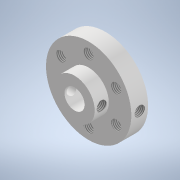
# Autodesk Inventor part: hub polulu
Saved by Autodesk Inventor 2020.3 (Build 243373000, 373)
## iProperties
Created: 2021-01-22
Part Number: hub polulu
Material: Generic
Document SubType Name: Modeling
Designer: Yu Jinyu
Density: 1 g/cm^3
Appearance: Default
Author: Yu Jinyu
Autodesk Inventor part; units mm, degrees
ref_plane "XZ Plane" through (0, 0, 0) normal (0, 1, 0) x (-1, 0, 0)
ref_plane "XY Plane" through (0, 0, 0) normal (0, 0, 1) x (1, 0, 0)
sketch "Sketch1" plane through (0, 0, 0) normal (0, 0, 1) x (1, 0, 0)
  circle A0 centre (0, 0) radius 12.7
  dimension "d0" = 25.4
  constraints: 1 centre point, 1 coincident
  measures "d0" diameter of A0
extrude "Extrusion1" add sketch "Sketch1" along normal blind 5
sketch "Sketch2" plane through (0, 0, 5) normal (0, 0, 1) x (1, 0, 0)
  circle A0 centre (0, 0) radius 6
  circle A1 centre (0, 0) radius 3
  dimension "d3" = 12
  dimension "d4" = 6
  constraints: 2 centre point, 2 coincident
  measures "d3" diameter of A0
  measures "d4" diameter of A1
extrude "Extrusion2" add sketch "Sketch2" along normal blind 4.2
sketch "Sketch3" plane through (0, 0, 5) normal (0, 0, 1) x (1, 0, 0)
  circle A0 centre (0, 0) radius 6 projected
  circle A1 centre (0, 0) radius 6
  circle A2 centre (0, 0) radius 9.5
  circle A3 centre (0, 9.5) radius 1.5
  circle A4 centre (0, 0) radius 3
  dimension "d7" = 19
  dimension "d8" = 3
  constraints: 3 centre point, 3 coincident, 1 vertical alignment, 2 other
  measures "d8" diameter of A3
extrude "Extrusion3" cut sketch "Sketch3" against normal blind 5 contours A3 A2 | A2 A3 | A4 picked at (0, 8.9912) picked at (0.0421, 9.9894)
pattern_circular "Circular Pattern1" count 6 over 360 about axis through (0, 0, 0) along (0, 0, 1) of "Extrusion1", "Extrusion3"
sketch "Sketch4" plane through (0, 0, 5) normal (0, 0, 1) x (1, 0, 0)
  circle A0 centre (0, 0) radius 9.5
  circle A1 centre (0, 9.5) radius 1.5
  dimension "d14" = 19
  dimension "d15" = 3
  constraints: 1 centre point, 1 coincident, 1 vertical alignment, 2 other
  measures "d15" diameter of A1
extrude "Extrusion4" cut sketch "Sketch4" against normal blind 10 contours A1 A0 | A0 A1 picked at (0, 8.9912) picked at (0.0421, 9.9894)
ref_plane "Work Plane1" through (12.7, 0, 0) normal (1, 0, 0) x (0, 1, 0)
sketch "Sketch6" plane through (12.7, 0, 0) normal (1, 0, 0) x (0, 1, 0)
  line L0 (0.693, 2.5) -> (-1.0754, 2.5)
  line L1 (12.7, 0) -> (-12.7, 0) projected
  circle A0 centre (-0.1912, 2.5) radius 1.5
  point P0 (0, 0)
  dimension "d19" = 2.5
  dimension "d20" = 3
  constraints: 2 end point, 1 centre point, 1 horizontal, 1 midpoint
  measures "d19" distance between parallel lines of L0 L1
  measures "d20" diameter of A0
extrude "Extrusion5" add sketch "Sketch6" against normal blind 25.4
sketch "Sketch7" plane through (12.7, 0, 0) normal (1, 0, 0) x (0, 1, 0)
  arc A0 (0, 1.0122) -> (0, 3.9878) centre (-0.1912, 2.5) ccw projected
  circle A1 centre (-0.1912, 2.5) radius 1.5
  circle A2 centre (0, 7.1) radius 1.5
  line L0 (6, 9.2) -> (-6, 9.2) projected
  point P0 (0, 0)
  point P1 (0, 3.9878)
  dimension "d23" = 3
  dimension "d24" = 2.1
  constraints: 1 centre point, 1 coincident, 3 other
  measures "d23" diameter of A2
  measures "d24" distance from line of L0 A2.centre
extrude "Extrusion6" cut sketch "Sketch7" against normal blind 25.4
thread "Thread1" size "M3x0.5" class "6H" standard "ANSI Metric M Profile" full length
thread "Thread2" size "M3x0.5" class "6H" standard "ANSI Metric M Profile" full length
thread "Thread3" size "M3x0.5" class "6H" standard "ANSI Metric M Profile" full length
thread "Thread4" size "M3x0.5" class "6H" standard "ANSI Metric M Profile" full length
thread "Thread5" size "M3x0.5" class "6H" standard "ANSI Metric M Profile" full length
thread "Thread6" size "M3x0.5" class "6H" standard "ANSI Metric M Profile" full length
thread "Thread7" size "M3x0.5" class "6H" standard "ANSI Metric M Profile" full length
thread "Thread9" size "M3x0.5" class "6H" standard "ANSI Metric M Profile" full length
thread "Thread11" size "M3x0.5" class "6H" standard "ANSI Metric M Profile" full length
thread "Thread12" size "M3x0.5" class "6H" standard "ANSI Metric M Profile" full length
body "Solid1"
